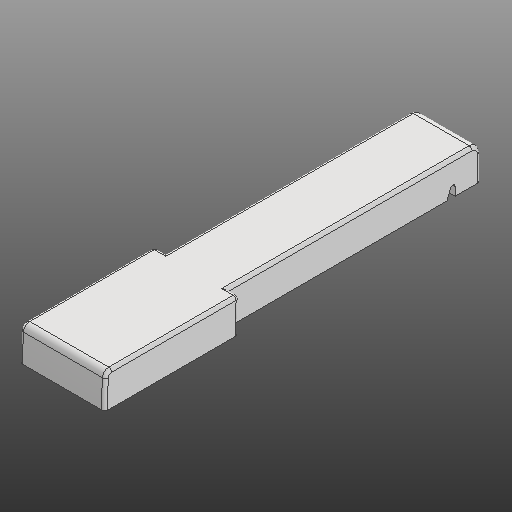
# Autodesk Inventor part: DKey0
Saved by Autodesk Inventor 2020 (Build 240168000, 168)
## iProperties
Created: 2019-12-01
Part Number: DKey0
Material: Generic
Document SubType Name: Modeling
Designer: Isaac Newcomb
Density: 1 g/cm^3
Appearance: Default
Mass: 11.7967 g
Surface Area: 48.5048 cm^2
Volume: 11.7967 cm^3
Project: Ice Keys
slotOffset: 1.047 mm
hingeRad: 0.500 mm
upperWidth: 14.600 mm
my_slotHeadOffset: 1.000 mm
my_slotHeadHeight: 3.000 mm
my_slotHeadWidth: 6.000 mm
my_neckSlotWidth: 4.300 mm
my_edgeSoftenRad: 0.700 mm
my_backWidth: 6.000 mm
my_hingeDepth: 2.000 mm
my_hingeCutRad: 0.570 mm
Author: Isaac Newcomb
Autodesk Inventor part; units mm, degrees
ref_plane "YZ Plane" through (0, 0, 0) normal (1, 0, 0) x (0, 1, 0)
ref_plane "XZ Plane" through (0, 0, 0) normal (0, 1, 0) x (-1, 0, 0)
ref_plane "Slot Start Plane" through (0, 0, -1.617) normal (0, 0, 1) x (1, 0, 0)
sketch "Key Profile" plane through (0, 0, 0) normal (1, 0, 0) x (0, 1, 0)
  line L0 (-2, 2.4306) -> (0.5472, 1.5035)
  arc A0 (1.2099, -1.047) -> (0.5472, 1.5035) centre (0, 0) ccw
  line L1 (-2, 1.3345) -> (0.195, 0.5356)
  arc A1 (0, -0.57) -> (0.195, 0.5356) centre (0, 0) ccw
  line L2 (-2, 2.4306) -> (-2, -0.57)
  line L3 (0, 0) -> (-2, 0) construction
  line L4 (0, -0.57) -> (-2, -0.57)
  line L5 (1.2099, -1.047) -> (-0.1005, -0.57)
  line L6 (6, -4.57) -> (6, 84.788)
  line L7 (-2, 84.9765) -> (-2, 2.4306)
  arc A2 (6, 84.788) -> (-2, 84.9765) centre (0, 0) ccw
  line L8 (-2, -0.57) -> (-2, -6.57)
  arc A3 (4, -6.57) -> (6, -4.57) centre (4, -4.57) ccw
  line L9 (-2, -6.57) -> (4, -6.57)
  arc A4 (6, 53.1625) -> (-2, 53.4626) centre (0, 0) ccw
  dimension "my_hingeCutRad" = 0.57
  dimension "my_hingeDepth" = 2
  dimension "my_hingeRegCutRad" = 1.6
  dimension "keyLength" = 85
  dimension "my_KeyHeight" = 8
  dimension "d107" = 20
  dimension "d122" = 4
  dimension "slotOffset" = 1.047
  dimension "my_backWidth" = 6
  dimension "d128" = 53.5
  constraints: 21 end point, 11 point on circle, 6 tangent, 5 centre point, 5 point on line, 4 coincident, 3 horizontal, 3 parallel, 2 vertical, 1 collinear
  measures "my_hingeCutRad" radius of A1
  measures "my_hingeDepth" distance of L3.start L3.end
  measures "my_hingeRegCutRad" radius of A0
  measures "keyLength" radius of A2
  measures "my_KeyHeight" distance from line of L6.start L7
  measures "d107" angle of L4 L1
  measures "d122" horizontal distance of A0.centre L9.end
  measures "slotOffset" vertical distance of L5.start point (0, 0)
  measures "my_backWidth" distance of L2.end L8.end
  measures "d128" radius of A4
extrude "Upper" add sketch "Key Profile" along normal mid plane 14.6 contours L7 A4 L6 A3 L9 L8 L4 L5 A0 L0 | L0 A0 L5 L4 A1 L1 L2
extrude "Lower" add sketch "Key Profile" along normal mid plane 20.0714 contours L7 A2 L6 A4
extrude "Protrusion Cutout" cut sketch "Key Profile" along normal mid plane 4.3 contours L0 A0 L5 L4 A1 L1 L2
fillet "Front Fillet" radius 1.5 1 edges at (0, 6, 84.788)
sketch "Slot Sketch" plane through (0, 0, -1.617) normal (0, 0, 1) x (1, 0, 0)
  line L0 (2.15, -2) -> (2.15, 1)
  line L1 (3, 4) -> (-3, 4)
  line L2 (-2.15, 1) -> (-2.15, -2)
  line L3 (-2.15, -2) -> (2.15, -2)
  line L4 (0, -2) -> (0, 4) construction
  line L5 (-3, 4) -> (-3, 1)
  line L6 (-3, 1) -> (-2.15, 1)
  line L7 (2.15, 1) -> (3, 1)
  line L8 (3, 1) -> (3, 4)
  point P0 (0, 0)
  dimension "d109" = 2
  dimension "my_slotHeadOffset" = 1
  dimension "my_slotHeadHeight" = 3
  dimension "my_slotHeadWidth" = 6
  dimension "my_neckSlotWidth" = 4.3
  constraints: 18 end point, 4 perpendicular, 3 parallel, 2 midpoint, 2 point on line, 2 vertical
  measures "d109" distance from line of point (0, 0) L3
  measures "my_slotHeadOffset" distance from line of L6 point (0, 0)
  measures "my_slotHeadHeight" distance of L1.end L5.end
  measures "my_slotHeadWidth" distance of L1.start L1.end
  measures "my_neckSlotWidth" distance of L2.end L0.start
extrude "Slot" cut sketch "Slot Sketch" against normal through all
fillet "Edge Softening" radius 0.7 16 edges at (7.3, 5.4142, -5.9842) (7.3, 1, -6.57) (7.3, 6, 24.2962) (-7.3, 5.4142, -5.9842) (-7.3, 1, -6.57) (-7.3, 6, 24.2962) (-10.0357, 5.5889, 84.4103) (-10.0357, 1.2914, 84.9902) (-10.0357, 6, 68.2706) (10.0357, 5.5889, 84.4103) (10.0357, 1.2914, 84.9902) (10.0357, 6, 68.2706) (-10.0357, 2.0056, 53.4624) (10.0357, 2.0056, 53.4624) (8.6679, 6, 53.1625) (-8.6679, 6, 53.1625)
equation "\"my_headHeight\" = 3"
equation "\"my_headOffset\" = 1"
equation "\"whiteKeyWidth\" = 20.07143"
body "Solid1"
